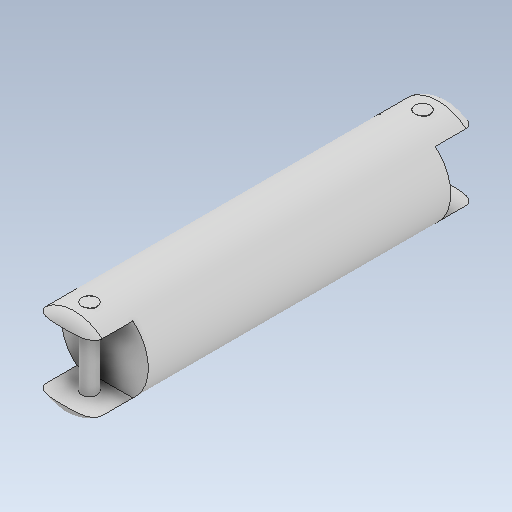
# Autodesk Inventor part: cylinder right
Saved by Autodesk Inventor 2021 (Build 250183000, 183)
## iProperties
Created: 2021-06-26
Part Number: cylinder right
Material: Generic
Document SubType Name: Modeling
Designer: TARUN
Density: 1 g/cm^3
Appearance: Default
Author: TARUN
Autodesk Inventor part; units mm, degrees
ref_plane "YZ Plane" through (0, 0, 0) normal (1, 0, 0) x (0, 1, 0)
ref_plane "XZ Plane" through (0, 0, 0) normal (0, 1, 0) x (-1, 0, 0)
ref_plane "XY Plane" through (0, 0, 0) normal (0, 0, 1) x (1, 0, 0)
sketch "Sketch1" plane through (0, 0, 0) normal (0, 0, 1) x (1, 0, 0)
  circle A0 centre (0, 0) radius 8.5
  dimension "d0" = 17
  constraints: 1 centre point, 1 coincident
  measures "d0" diameter of A0
extrude "Extrusion1" add sketch "Sketch1" along normal blind 75
sketch "Sketch2" plane through (0, 0, 0) normal (0, 1, 0) x (-1, 0, 0)
  circle A0 centre (0, 70) radius 1.5
  line L0 (8.5, 75) -> (-8.5, 75) projected
  circle A1 centre (0, 5) radius 1.5
  line L1 (8.5, 0) -> (-8.5, 0) projected
  point P0 (0, 0)
  dimension "d3" = 3
  dimension "d4" = 5
  dimension "d5" = 3
  dimension "d6" = 5
  constraints: 2 centre point
  measures "d3" diameter of A0
  measures "d4" distance from line of L0 A0.centre
  measures "d5" diameter of A1
  measures "d6" distance from line of L1 A1.centre
extrude "Extrusion2" cut sketch "Sketch2" against normal through all both and the other way through all
fillet "Fillet1" radius 2 2 edges at (-8.5, 0, 75) (-8.5, 0, 0)
sketch "Sketch5" plane through (0, 0, 75) normal (0, 0, 1) x (1, 0, 0)
  line L0 (-16.9, 6.5) -> (17, 6.5)
  line L1 (17, 6.5) -> (17, -6.5)
  line L2 (17, -6.5) -> (-16.9, -6.5)
  line L3 (-16.9, -6.5) -> (-16.9, 6.5)
  point P0 (0, 0)
  dimension "d18" = 13
  dimension "d19" = 6.5
  constraints: 8 end point, 2 parallel, 1 horizontal, 1 perpendicular
  measures "d18" distance between parallel lines of L2 L0
  measures "d19" distance from line of point (0, 0) L0
extrude "Extrusion5" cut sketch "Sketch5" against normal blind 8
sketch "Sketch6" plane through (0, 0, 0) normal (0, 0, -1) x (-1, 0, 0)
  line L0 (-15.4684, 6.5) -> (16.538, 6.5)
  line L1 (16.538, 6.5) -> (16.538, -6.5)
  line L2 (16.538, -6.5) -> (-15.4684, -6.5)
  line L3 (-15.4684, -6.5) -> (-15.4684, 6.5)
  point P0 (0, 0)
  dimension "d22" = 13
  dimension "d23" = 6.5
  constraints: 8 end point, 2 parallel, 1 horizontal, 1 perpendicular
  measures "d22" distance between parallel lines of L2 L0
  measures "d23" distance from line of point (0, 0) L0
extrude "Extrusion6" cut sketch "Sketch6" against normal blind 8
sketch "Sketch7" plane through (-5.4772, -6.5, 8) normal (0, 1, 0) x (1, 0, 0)
  circle A0 centre (5.4772, 3) radius 1.5 projected
  line L0 (10.9545, -59) -> (0, -59) projected
  line L1 (0, -65) -> (0, -59) projected
  line L2 (10.9545, -59) -> (10.9545, -65) projected
  line L3 (10.9545, 0) -> (10.9545, -59) projected
  line L4 (0, 0) -> (10.9545, 0) projected
  line L5 (0, 0) -> (0, 6) projected
  line L6 (10.9545, 6) -> (10.9545, 0) projected
  line L7 (0, -59) -> (0, 0) projected
  circle A1 centre (5.4772, -62) radius 1.5 projected
  point P0 (5.4772, 8)
  point P1 (5.4772, -67)
  constraints: 4 other
extrude "Extrusion7" add sketch "Sketch7" along normal blind 15 and the other way blind 2 contours A0
sketch "Sketch8" plane through (-5.4772, 6.5, 67) normal (0, -1, 0) x (1, 0, 0)
  circle A0 centre (5.4772, -62) radius 1.5 projected
  line L0 (0, 0) -> (10.9545, 0) projected
  line L1 (10.9545, 6) -> (10.9545, 0) projected
  line L2 (0, 0) -> (0, 6) projected
  line L3 (0, -59) -> (0, 0) projected
  line L4 (10.9545, -59) -> (0, -59) projected
  line L5 (10.9545, -59) -> (10.9545, -65) projected
  line L6 (0, -65) -> (0, -59) projected
  line L7 (10.9545, 0) -> (10.9545, -59) projected
  circle A1 centre (5.4772, 3) radius 1.5 projected
  point P0 (5.4772, -67)
  point P1 (5.4772, 8)
  constraints: 4 other
extrude "Extrusion8" add sketch "Sketch8" along normal blind 15 and the other way blind 2 contours A1
body "Solid1"
